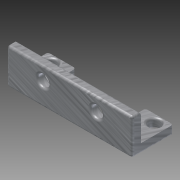
# Autodesk Inventor part: Stepper_Bracket
Saved by Autodesk Inventor 2012 (Build 160160000, 160)
## iProperties
Created: 2012-10-05
Part Number: Stepper_Bracket
Material: Default
Document SubType Name: Modeling
Designer: agmeyer
Density: 1 g/cm^3
Author: agmeyer
Autodesk Inventor part; units mm, degrees
ref_plane "YZ Plane" through (0, 0, 0) normal (1, 0, 0) x (0, 1, 0)
ref_plane "XZ Plane" through (0, 0, 0) normal (0, 1, 0) x (-1, 0, 0)
ref_plane "XY Plane" through (0, 0, 0) normal (0, 0, 1) x (1, 0, 0)
sketch "Sketch1" plane through (0, 0, 0) normal (0, 0, 1) x (1, 0, 0)
  line L0 (-13.97, 4.6) -> (-13.97, -4.6)
  line L1 (-13.97, -4.6) -> (13.97, -4.6)
  line L2 (13.97, -4.6) -> (13.97, 4.6)
  line L3 (13.97, 4.6) -> (7.77, 4.6)
  line L4 (-13.97, 4.6) -> (-7.77, 4.6)
  line L5 (-13.97, 4.6) -> (13.97, -4.6) construction
  line L6 (13.97, 4.6) -> (-13.97, -4.6) construction
  line L7 (-7.77, 4.6) -> (-7.77, -2.6)
  line L8 (-7.77, -2.6) -> (7.77, -2.6)
  line L9 (7.77, -2.6) -> (7.77, 4.6)
  point P0 (0, 0)
  point P1 (0, 0)
  dimension "d1" = 27.94
  dimension "d3" = 6.2
  dimension "d5" = 9.2
  dimension "d6" = 7.2
  constraints: 20 end point, 4 midpoint, 4 perpendicular, 2 collinear, 2 parallel, 1 vertical
  measures "d1" distance of L0.end L1.end
  measures "d3" distance of L0.start L4.end
  measures "d5" distance between parallel lines of L1 L3
  measures "d6" distance between parallel lines of L3 L8
extrude "Extrusion1" add sketch "Sketch1" along normal blind 2
sketch "Sketch2" plane through (0, 0, 2) normal (0, 0, 1) x (1, 0, 0)
  line L0 (13.97, 4.6) -> (13.97, -4.6) projected
  line L1 (-7.77, -2.6) -> (7.77, -2.6) projected
  line L2 (-13.97, -4.6) -> (13.97, -4.6)
  line L3 (13.97, -4.6) -> (13.97, -2.6)
  line L4 (13.97, -2.6) -> (-13.97, -2.6)
  line L5 (-13.97, -2.6) -> (-13.97, -4.6)
  point P0 (0, 0)
  constraints: 8 end point, 2 parallel, 1 collinear, 1 horizontal, 1 perpendicular, 1 point on line
extrude "Extrusion2" add sketch "Sketch2" along normal blind 6
hole "Hole3" at (-5.97, -2.6, 5) direction (0, -1, 0) diameter 2.5 end through all
hole "Hole4" at (5.97, -2.6, 5) direction (0, -1, 0) diameter 2.5 end through all
sketch "Sketch3" plane through (0, 0, 2) normal (0, 0, 1) x (1, 0, 0)
  line L0 (-13.97, -2.6) -> (-13.97, 4.6) projected
  line L1 (-11.557, 2.9) -> (11.557, 2.9) construction
  line L2 (-13.97, -2.6) -> (13.97, -2.6) construction
  line L3 (0, 0) -> (0, 2.9) construction
  dimension "d47" = 23.114
  dimension "d48" = 5.5
  constraints: 4 end point, 2 perpendicular, 1 midpoint, 1 parallel
  measures "d47" distance of L1.start L1.end
  measures "d48" distance between parallel lines of L2 L1
hole "Hole5" at (-11.557, 2.9, 2) at (11.557, 2.9, 2) direction (0, 0, -1) diameter 2.5 end through all
fillet "Fillet1" radius 0.5 21 edges at (-11.557, 4.15, 0) (-11.557, 4.15, 2) (-5.97, -2.6, 3.75) (-5.97, -4.6, 3.75) (11.557, 4.15, 2) (11.557, 4.15, 0) (5.97, -2.6, 3.75) (5.97, -4.6, 3.75) (-13.97, 4.6, 1) (-7.77, 4.6, 1) (7.77, 4.6, 1) (13.97, 4.6, 1) (13.97, 0, 0) (13.97, -4.6, 4) (13.97, -3.6, 8) (-13.97, -3.6, 8) (-13.97, -4.6, 4) (0, -4.6, 0) (-13.97, 0, 0) (0, -4.6, 8) (0, -2.6, 8)
body "Solid1"
